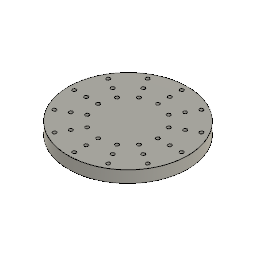
Circular tube cartridge v5 (Autodesk Fusion 360 design; units mm, degrees)
Autodesk Fusion 360 part; units mm, degrees
sketch "base plate" plane through (0, 0, 0) normal (0, 0, 1) x (1, 0, 0)
  circle A0 centre (0, 0) radius 50
  dimension "d1" = 100
  constraint coincident A0.centre origin
  measures "d1" diameter of A0
extrude "Extrude1" add sketch "base plate" along normal mid plane 10
sketch "tube holes outer layer" plane through (0, 0, 5) normal (0, 0, 1) x (-1, 0, 0)
  circle A0 centre (0, 0) radius 50
  circle A1 centre (45, 0) radius 1.5
  point P0 (-45, 0)
  point P1 (-38.9711, -22.5)
  point P2 (-22.5, -38.9711)
  point P3 (0, -45)
  point P4 (22.5, -38.9711)
  point P5 (38.9711, -22.5)
  point P6 (38.9711, 22.5)
  point P7 (22.5, 38.9711)
  point P8 (0, 45)
  point P9 (-22.5, 38.9711)
  point P10 (-38.9711, 22.5)
  dimension "d4" = 3
  dimension "d6" = 360
  measures "d4" diameter of A1
hole "Hole1" at (0, 45, 5) at (22.5, 38.9711, 5) at (38.9711, 22.5, 5) at (45, 0, 5) at (38.9711, -22.5, 5) at (22.5, -38.9711, 5) at (0, -45, 5) at (-22.5, -38.9711, 5) at (-38.9711, -22.5, 5) at (-45, 0, 5) at (-38.9711, 22.5, 5) at (-22.5, 38.9711, 5) direction (0, 0, -1) diameter 3 depth 9 tip angle 118
sketch "tube holes layer 2" plane through (0, 0, 5) normal (0, 0, 1) x (-1, 0, 0)
  circle A0 centre (38.9711, -22.5) radius 1.5
  circle A1 centre (38.9711, 22.5) radius 1.5
  circle A2 centre (0, 45) radius 1.5
  circle A3 centre (-38.9711, 22.5) radius 1.5
  circle A4 centre (-38.9711, -22.5) radius 1.5
  circle A5 centre (0, -45) radius 1.5
  circle A6 centre (-22.5, -38.9711) radius 1.5
  circle A7 centre (-45, 0) radius 1.5
  circle A8 centre (-22.5, 38.9711) radius 1.5
  circle A9 centre (22.5, 38.9711) radius 1.5
  circle A10 centre (45, 0) radius 1.5
  circle A11 centre (22.5, -38.9711) radius 1.5
  circle A12 centre (0, 0) radius 50
  line L0 (0, 0) -> (0, -45) construction
  circle A13 centre (0, -35) radius 1.5
  circle A14 centre (0, 35) radius 1.5
  circle A15 centre (-17.5, 30.3109) radius 1.5
  circle A16 centre (-30.3109, 17.5) radius 1.5
  circle A17 centre (-35, 0) radius 1.5
  circle A18 centre (-30.3109, -17.5) radius 1.5
  circle A19 centre (-17.5, -30.3109) radius 1.5
  circle A20 centre (17.5, -30.3109) radius 1.5
  circle A21 centre (30.3109, -17.5) radius 1.5
  circle A22 centre (35, 0) radius 1.5
  circle A23 centre (30.3109, 17.5) radius 1.5
  circle A24 centre (17.5, 30.3109) radius 1.5
  dimension "d10" = 3
  dimension "d12" = 360
  constraint coincident A12.centre L0.start
  constraint coincident A5.centre L0.end
  constraint coincident L0 A13.centre
  measures "d10" diameter of A13
hole "Hole2" at (-17.5, 30.3109, 5) at (0, 35, 5) at (17.5, 30.3109, 5) at (30.3109, 17.5, 5) at (35, 0, 5) at (30.3109, -17.5, 5) at (17.5, -30.3109, 5) at (0, -35, 5) at (-17.5, -30.3109, 5) at (-30.3109, -17.5, 5) at (-35, 0, 5) at (-30.3109, 17.5, 5) direction (0, 0, -1) diameter 3 depth 9 tip angle 118
sketch "tube holes layer 3" plane through (0, 0, 5) normal (0, 0, 1) x (-1, 0, 0)
  circle A0 centre (35, 0) radius 1.5
  circle A1 centre (17.5, 30.3109) radius 1.5
  circle A2 centre (-17.5, 30.3109) radius 1.5
  circle A3 centre (-35, 0) radius 1.5
  circle A4 centre (-17.5, -30.3109) radius 1.5
  circle A5 centre (17.5, -30.3109) radius 1.5
  circle A6 centre (0, -35) radius 1.5
  circle A7 centre (-30.3109, -17.5) radius 1.5
  circle A8 centre (-30.3109, 17.5) radius 1.5
  circle A9 centre (0, 35) radius 1.5
  circle A10 centre (30.3109, 17.5) radius 1.5
  circle A11 centre (30.3109, -17.5) radius 1.5
  circle A12 centre (38.9711, -22.5) radius 1.5
  circle A13 centre (38.9711, 22.5) radius 1.5
  circle A14 centre (0, 45) radius 1.5
  circle A15 centre (-38.9711, 22.5) radius 1.5
  circle A16 centre (-38.9711, -22.5) radius 1.5
  circle A17 centre (0, -45) radius 1.5
  circle A18 centre (-22.5, -38.9711) radius 1.5
  circle A19 centre (-45, 0) radius 1.5
  circle A20 centre (-22.5, 38.9711) radius 1.5
  circle A21 centre (22.5, 38.9711) radius 1.5
  circle A22 centre (45, 0) radius 1.5
  circle A23 centre (22.5, -38.9711) radius 1.5
  circle A24 centre (0, 0) radius 50
  circle A25 centre (0, -25) radius 1.5
  point P0 (0, 25)
  point P1 (-12.5, 21.6506)
  point P2 (-21.6506, 12.5)
  point P3 (-25, 0)
  point P4 (-21.6506, -12.5)
  point P5 (-12.5, -21.6506)
  point P6 (12.5, -21.6506)
  point P7 (21.6506, -12.5)
  point P8 (25, 0)
  point P9 (21.6506, 12.5)
  point P10 (12.5, 21.6506)
  dimension "d16" = 3
  dimension "d18" = 360
  measures "d16" diameter of A25
hole "Hole3" at (0, 25, 5) at (12.5, 21.6506, 5) at (21.6506, 12.5, 5) at (25, 0, 5) at (21.6506, -12.5, 5) at (12.5, -21.6506, 5) at (0, -25, 5) at (-12.5, -21.6506, 5) at (-21.6506, -12.5, 5) at (-25, 0, 5) at (-21.6506, 12.5, 5) at (-12.5, 21.6506, 5) direction (0, 0, -1) diameter 3 depth 9 tip angle 118
